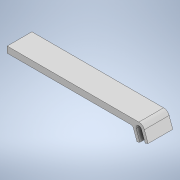
# Autodesk Inventor part: grip_N_fix
Saved by Autodesk Inventor 2021 (Build 250183000, 183)
## iProperties
Created: 2021-05-09
Part Number: grip_N_fix
Material: Generic
Document SubType Name: Modeling
Designer: Alsayaary
Density: 1 g/cm^3
Appearance: Default
Author: Abdulrahman
Autodesk Inventor part; units mm, degrees
ref_plane "YZ Plane" through (0, 0, 0) normal (1, 0, 0) x (0, 1, 0)
ref_plane "XZ Plane" through (0, 0, 0) normal (0, 1, 0) x (-1, 0, 0)
ref_plane "XY Plane" through (0, 0, 0) normal (0, 0, 1) x (1, 0, 0)
sketch "Sketch1" plane through (0, 0, 0) normal (0, 0, 1) x (1, 0, 0)
  line L0 (182.3, 94.0782) -> (194.1165, 61.6124)
  line L1 (194.1165, 61.6124) -> (203.5135, 65.0326)
  line L2 (203.5135, 65.0326) -> (191.5428, 97.9218)
  arc A0 (208.4572, 104.0782) -> (191.5428, 97.9218) centre (200, 101) ccw
  line L3 (208.4572, 104.0782) -> (220.4279, 71.1889)
  line L4 (220.4279, 71.1889) -> (229.8249, 74.6091)
  line L5 (229.8249, 74.6091) -> (217.8542, 107.4984)
  arc A1 (217.8542, 107.4984) -> (200, 120) centre (200, 101) ccw
  line L6 (173.8427, 100) -> (-226.1573, 100)
  line L7 (200, 120) -> (-226.1573, 120)
  line L8 (-226.1573, 120) -> (-226.1573, 100)
  line L9 (0, 135.0552) -> (0, 49.3719) projected
  line L10 (-317.3537, 0) -> (321.0213, 0) projected
  arc A2 (182.3, 94.0782) -> (173.8427, 100) centre (173.8427, 91) ccw
  dimension "d38" = 10
  dimension "d39" = 10
  dimension "d40" = 9
  dimension "d47" = 20
  dimension "d53" = 9
  dimension "d56" = 400
  dimension "d58" = 200
  dimension "d59" = 35
  dimension "d60" = 20
  dimension "d61" = 100
  constraints: 18 end point, 6 perpendicular, 6 point on circle, 6 tangent, 3 centre point, 1 coincident, 1 collinear, 1 parallel
  measures "d38" distance of L3.end L4.end
  measures "d39" distance of L0.end L1.end
  measures "d40" radius of A0
  measures "d47" distance of L7.end L6.end
  measures "d53" radius of A2
  measures "d56" distance of L6.start L6.end
  measures "d58" distance from line of L9 A0.centre
  measures "d59" distance from line of A0.centre L4
  measures "d60" angle of L1 L6
  measures "d61" distance between parallel lines of L10 L6
extrude "Extrusion1" add sketch "Sketch1" along normal mid plane 80
equation "\"d39\" = d38"
equation "\"secure_arm_radii\" = 9"
equation "\"secure_arm_hold_length\" = 35"
equation "\"rack_tooth_thickness\" = 5"
equation "\"rack_tooth_addendum\" = 5"
equation "\"rack_tooth_dedendum\" = 5"
equation "\"hoop_bearing_length\" = 5deg"
equation "\"secure_arm_angle\" = 20deg"
equation "\"hoop_tabs_thickness\" = 6"
equation "\"hoop_tabs_hole\" = 4"
equation "\"support_baseClamp_thickness\" = 8"
equation "\"support_frame_endHoleBuffer\" = 25"
equation "\"support_frame_squareBarThickness\" = 5"
equation "\"support_baseClamp_sleeveSweepTerminationAngle\" = 55deg"
equation "\"support_baseClamp_sleeveHoleDiameter\" = 12"
equation "\"support_frame_squareBarFillet\" = 2"
equation "\"support_baseClamp_platformWidthBuffer\" = 0"
equation "\"support_baseClamp_platformThickness\" = 15"
equation "\"support_baseClamp_platformLengthBuffer\" = 35"
equation "\"hoop_angle_z\" = 45deg"
equation "\"hoop_cable_diam\" = 5"
equation "\"hoop_cable_pulley_diam\" = 22"
body "Solid1"
